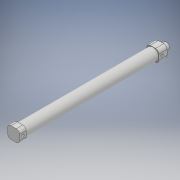
# Autodesk Inventor part: SMC_CJ2B16-175(本体)
Saved by Autodesk Inventor 2018 (Build 220112000, 112)
## iProperties
Created: 2018-04-28
Part Number: SMC_CJ2B16-175(本体)
Material: 一般
Document SubType Name: Modeling
Designer: Take
Density: 1 g/cm^3
Appearance: 既定
Author: Take
Autodesk Inventor part; units mm, degrees
ref_plane "YZ Plane" through (0, 0, 0) normal (1, 0, 0) x (0, 1, 0)
ref_plane "XZ Plane" through (0, 0, 0) normal (0, 1, 0) x (-1, 0, 0)
ref_plane "XY Plane" through (0, 0, 0) normal (0, 0, 1) x (1, 0, 0)
sketch "スケッチ1" plane through (0, 0, 0) normal (0, 1, 0) x (-1, 0, 0)
  line L0 (-4, -9) -> (4, -9)
  line L1 (9, -4) -> (9, 4)
  line L2 (4, 9) -> (-4, 9)
  line L3 (-9, 4) -> (-9, -4)
  arc A0 (9, 4) -> (4, 9) centre (4, 4) ccw
  arc A1 (-4, 9) -> (-9, 4) centre (-4, 4) ccw
  arc A2 (-9, -4) -> (-4, -9) centre (-4, -4) ccw
  arc A3 (4, -9) -> (9, -4) centre (4, -4) ccw
  point P0 (0, 0)
  point P1 (9, 0)
  point P2 (0, -9)
  point P3 (9, 4)
  point P4 (9, -4)
  point P5 (4, 9)
  point P6 (-4, 9)
  point P7 (-9, -4)
  point P8 (4, -9)
  dimension "d0" = 5
  constraints: 8 end point, 8 point on circle, 8 point on line, 8 tangent, 4 centre point, 3 equal radius, 2 parallel, 1 horizontal, 1 perpendicular
  measures "d0" radius of A0
extrude "押し出し1" add sketch "スケッチ1" along normal blind 10
sketch "スケッチ2" plane through (0, 10, 0) normal (0, 1, 0) x (1, 0, 0)
  circle A0 centre (0, 0) radius 8.7
  dimension "d3" = 17.4
  constraints: 1 centre point, 1 coincident
  measures "d3" diameter of A0
extrude "押し出し2" add sketch "スケッチ2" along normal blind 200
sketch "スケッチ3" plane through (0, 210, 0) normal (0, 1, 0) x (1, 0, 0)
  point P0 (0, 0)
sketch "スケッチ4" plane through (0, 210, 0) normal (0, 1, 0) x (1, 0, 0)
  line L0 (-4, 9) -> (4, 9)
  line L1 (4, 9) -> (-4, 9) projected
  line L2 (9, 4) -> (9, -4)
  line L3 (4, -9) -> (-4, -9)
  line L4 (-9, -4) -> (-9, 4)
  arc A0 (-9, -4) -> (-4, -9) centre (-4, -4) ccw
  arc A1 (-4, 9) -> (-9, 4) centre (-4, 4) ccw
  arc A2 (9, 4) -> (4, 9) centre (4, 4) ccw
  arc A3 (4, -9) -> (9, -4) centre (4, -4) ccw
  point P0 (0, 0)
  point P1 (-9, 9)
  point P2 (9, 9)
  dimension "d6" = 18
  dimension "d7" = 5
  constraints: 8 end point, 8 point on circle, 8 tangent, 4 centre point, 4 point on line, 3 equal radius, 3 perpendicular, 1 collinear
  measures "d6" distance of point (-9, 9) point (9, 9)
  measures "d7" radius of A0
extrude "押し出し3" add sketch "スケッチ4" along normal blind 12.4
sketch "スケッチ5" plane through (0, 222.4, 0) normal (0, 1, 0) x (1, 0, 0)
  circle A0 centre (0, 0) radius 5
  dimension "d10" = 10
  constraints: 1 centre point, 1 coincident
  measures "d10" diameter of A0
extrude "押し出し4" add sketch "スケッチ5" along normal blind 8
sketch "スケッチ6" plane through (0, 230.4, 0) normal (0, 1, 0) x (1, 0, 0)
  circle A0 centre (0, 0) radius 2.5
  dimension "d13" = 5
  constraints: 2 coincident, 1 centre point
  measures "d13" diameter of A0
extrude "押し出し5" cut sketch "スケッチ6" against normal blind 180
sketch "スケッチ7" plane through (9, 0, 4) normal (1, 0, 0) x (0, 0, -1)
  line L0 (4, 0) -> (4, 10)
  line L1 (0, 10) -> (8, 10) projected
  circle A0 centre (4, 5) radius 2
  dimension "d16" = 4
  constraints: 2 end point, 2 midpoint, 1 centre point, 1 coincident
  measures "d16" diameter of A0
extrude "押し出し6" cut sketch "スケッチ7" against normal blind 11.6
sketch "スケッチ8" plane through (9, 210, 4) normal (1, 0, 0) x (0, 0, -1)
  line L0 (0, 0) -> (8, 0) projected
  line L1 (4, 0) -> (4, 12.4)
  line L2 (-1, 12.4) -> (9, 12.4) projected
  circle A0 centre (4, 4.5) radius 2
  point P0 (4, -210)
  dimension "d19" = 4.5
  dimension "d20" = 4
  constraints: 2 end point, 2 midpoint, 1 centre point, 1 coincident, 1 point on line
  measures "d19" distance from line of L0 point (4, 4.5)
  measures "d20" diameter of A0
extrude "押し出し7" cut sketch "スケッチ8" against normal blind 6.9
